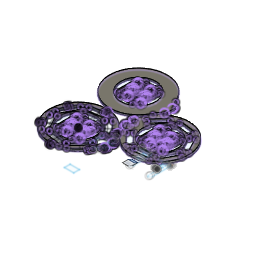
plywood_lamp (Autodesk Fusion 360 design; units mm, degrees)
Autodesk Fusion 360 part; units mm, degrees
(part 1 of 2)
sketch "Sketch1" plane through (0, 0, 0) normal (0, 1, 0) x (1, 0, 0)
  circle A0 centre (0, 0) radius 32
  circle A1 centre (0, 0) radius 52.5
  line L0 (34, 9.25) -> (57, 9.25)
  line L1 (57, 9.25) -> (57, -9.25)
  line L2 (57, -9.25) -> (34, -9.25)
  line L3 (34, -9.25) -> (34, 9.25)
  line L4 (50, 4.3983) -> (59, 4.3983)
  line L5 (59, 4.3983) -> (59, -4.6017)
  line L6 (59, -4.6017) -> (50, -4.6017)
  line L7 (50, -4.6017) -> (50, 4.3983)
  line L8 (50, -65) -> (67, -65)
  line L9 (67, -65) -> (67, -75.4)
  line L10 (67, -75.4) -> (50, -75.4)
  line L11 (50, -75.4) -> (50, -65)
  line L12 (0, 0) -> (34, 0)
  line L13 (0, 0) -> (25.0674, -22.9701)
  line L14 (25.0674, -22.9701) -> (36.5525, -10.4364)
  line L15 (36.5525, -10.4364) -> (44.2201, -17.4625)
  line L16 (44.2201, -17.4625) -> (32.7351, -29.9962)
  line L17 (32.7351, -29.9962) -> (25.0674, -22.9701)
  line L18 (25.0674, -22.9701) -> (13.5824, -35.5038)
  line L19 (13.5824, -35.5038) -> (21.2501, -42.5299)
  line L20 (21.2501, -42.5299) -> (32.7351, -29.9962)
  line L21 (32.7351, -29.9962) -> (25.0674, -22.9701)
  line L22 (0, 0) -> (-4.4379, -33.7091)
  line L23 (-5.7954, -44.0202) -> (-4.4379, -33.7091)
  line L24 (-4.4379, -33.7091) -> (12.4167, -35.9281)
  line L25 (11.0592, -46.2391) -> (-5.7954, -44.0202)
  line L26 (12.4167, -35.9281) -> (11.0592, -46.2391)
  line L27 (-4.4379, -33.7091) -> (-21.2925, -31.4902)
  line L28 (-22.6499, -41.8012) -> (-5.7954, -44.0202)
  line L29 (-21.2925, -31.4902) -> (-22.6499, -41.8012)
  line L30 (0, 0) -> (-30.1584, -15.6995)
  line L31 (-39.3833, -20.5016) -> (-30.1584, -15.6995)
  line L32 (-30.1584, -15.6995) -> (-22.3086, -30.7786)
  line L33 (-31.5336, -35.5808) -> (-39.3833, -20.5016)
  line L34 (-22.3086, -30.7786) -> (-31.5336, -35.5808)
  line L35 (-30.1584, -15.6995) -> (-38.0081, -0.6203)
  line L36 (-47.233, -5.4225) -> (-39.3833, -20.5016)
  line L37 (-38.0081, -0.6203) -> (-47.233, -5.4225)
  line L38 (0, 0) -> (-30.1584, 15.6995)
  line L39 (-39.3833, 20.5016) -> (-30.1584, 15.6995)
  line L40 (-30.1584, 15.6995) -> (-38.0081, 0.6203)
  line L41 (-47.233, 5.4225) -> (-39.3833, 20.5016)
  line L42 (-38.0081, 0.6203) -> (-47.233, 5.4225)
  line L43 (-30.1584, 15.6995) -> (-22.3086, 30.7786)
  line L44 (-31.5336, 35.5808) -> (-39.3833, 20.5016)
  line L45 (-22.3086, 30.7786) -> (-31.5336, 35.5808)
  line L46 (0, 0) -> (-4.4379, 33.7091)
  line L47 (-5.7954, 44.0202) -> (-4.4379, 33.7091)
  line L48 (-4.4379, 33.7091) -> (-21.2925, 31.4902)
  line L49 (-22.6499, 41.8012) -> (-5.7954, 44.0202)
  line L50 (-21.2925, 31.4902) -> (-22.6499, 41.8012)
  line L51 (-4.4379, 33.7091) -> (12.4167, 35.9281)
  line L52 (11.0592, 46.2391) -> (-5.7954, 44.0202)
  line L53 (12.4167, 35.9281) -> (11.0592, 46.2391)
  line L54 (0, 0) -> (25.0674, 22.9701)
  line L55 (32.7351, 29.9962) -> (25.0674, 22.9701)
  line L56 (25.0674, 22.9701) -> (13.5824, 35.5038)
  line L57 (21.2501, 42.5299) -> (32.7351, 29.9962)
  line L58 (13.5824, 35.5038) -> (21.2501, 42.5299)
  line L59 (25.0674, 22.9701) -> (36.5525, 10.4364)
  line L60 (44.2201, 17.4625) -> (32.7351, 29.9962)
  line L61 (36.5525, 10.4364) -> (44.2201, 17.4625)
  circle A2 centre (0, 0) radius 38.0132
  circle A3 centre (0, 0) radius 47.5432
  line L62 (55, 12.25) -> (34, 12.25)
  line L63 (34, 12.25) -> (34, -12.25)
  line L64 (34, -12.25) -> (55, -12.25)
  line L65 (60, -7.25) -> (60, 7.25)
  arc A4 (55, -12.25) -> (60, -7.25) centre (55, -7.25) ccw
  arc A5 (60, 7.25) -> (55, 12.25) centre (55, 7.25) ccw
  spline S0 degree 5 poles (58.5355, -10.7855) (58.375, -10.946) (58.0274, -11.2549) (57.426, -11.6816) (56.4828, -12.1897) (55.1674, -12.7909) (53.8333, -13.4415) (52.5876, -14.2222) (51.4896, -15.1867) (50.5348, -16.3509) (49.6862, -17.7123) (49.0515, -18.9501) (48.5799, -19.957) (48.2645, -20.6625) (48.1066, -21.0238) knots 0 0 0 0 0 0 0.1 0.2 0.3 0.4 0.5 0.6 0.7 0.8 0.9 1 1 1 1 1 1
  line L66 (59.4934, -9.8277) -> (57.5777, -11.7434)
  line L67 (48.9119, -19.1812) -> (47.3014, -22.8664)
  spline S1 degree 5 poles (58.5355, 10.7855) (58.3764, 10.9446) (58.0317, 11.2507) (57.4349, 11.6734) (56.4973, 12.1769) (55.1846, 12.7765) (53.845, 13.4321) (52.5838, 14.2253) (51.463, 15.2079) (50.4859, 16.3894) (49.6261, 17.7595) (48.9998, 18.9905) (48.5482, 19.9817) (48.2529, 20.6716) (48.1066, 21.0238) knots 0 0 0 0 0 0 0.1 0.2 0.3 0.4 0.5 0.6 0.7 0.8 0.9 1 1 1 1 1 1
  line L68 (59.4849, 9.8361) -> (57.5861, 11.7349)
  line L69 (48.851, 19.231) -> (47.3623, 22.8167)
  spline S2 degree 5 poles (57, -9.25) (56.1534, -9.25) (54.5378, -9.3901) (52.3465, -10.0199) (49.8421, -11.547) (47.2933, -13.9608) (45.7147, -15.761) (44.8358, -16.7778) (44.4003, -17.2659) (44.2201, -17.4625) knots 0 0 0 0 0 0 0.2 0.4 0.6 0.8 1 1 1 1 1 1
  line L70 (59, -9.25) -> (55, -9.25)
  line L71 (44.672, -16.9694) -> (43.7683, -17.9556)
  spline S3 degree 5 poles (57, 9.25) (56.1534, 9.25) (54.557, 9.3691) (52.452, 9.9048) (50.1458, 11.2155) (47.8255, 13.38) (46.2557, 15.1706) (45.1945, 16.3864) (44.5366, 17.1171) (44.2201, 17.4625) knots 0 0 0 0 0 0 0.2 0.4 0.6 0.8 1 1 1 1 1 1
  line L72 (59, 9.25) -> (55, 9.25)
  line L73 (45.0141, 16.5961) -> (43.4262, 18.3289)
  line L74 (59, 4.3983) -> (60, 4.3983)
  line L75 (59, -4.6017) -> (60, -4.6017)
  line L76 (0, 0) -> (45.4663, -26.25)
  line L77 (41.1362, -23.75) -> (42.0112, -22.2345)
  line L78 (42.0112, -22.2345) -> (46.3161, -24.7199)
  line L79 (41.1362, -23.75) -> (40.2612, -25.2655)
  line L80 (40.2612, -25.2655) -> (44.5661, -27.751)
  line L81 (0, 0) -> (45.4663, 26.25)
  line L82 (40.2612, 25.2655) -> (44.5661, 27.751)
  line L83 (42.0112, 22.2345) -> (46.3161, 24.7199)
  line L84 (41.1362, 23.75) -> (42.0112, 22.2345)
  line L85 (41.1362, 23.75) -> (40.2612, 25.2655)
  line L86 (0, 0) -> (0, 52.5)
  line L87 (-1.75, 47.5) -> (-1.75, 52.4708)
  line L88 (1.75, 47.5) -> (1.75, 52.4708)
  line L89 (0, 47.5) -> (1.75, 47.5)
  line L90 (0, 47.5) -> (-1.75, 47.5)
  line L91 (0, 0) -> (-45.4663, 26.25)
  line L92 (-42.0112, 22.2345) -> (-46.3161, 24.7199)
  line L93 (-40.2612, 25.2655) -> (-44.5661, 27.751)
  line L94 (-41.1362, 23.75) -> (-40.2612, 25.2655)
  line L95 (-41.1362, 23.75) -> (-42.0112, 22.2345)
  line L96 (0, 0) -> (-45.4663, -26.25)
  line L97 (-40.2612, -25.2655) -> (-44.5661, -27.751)
  line L98 (-42.0112, -22.2345) -> (-46.3161, -24.7199)
  line L99 (-41.1362, -23.75) -> (-42.0112, -22.2345)
  line L100 (-41.1362, -23.75) -> (-40.2612, -25.2655)
  line L101 (0, 0) -> (0, -52.5)
  line L102 (1.75, -47.5) -> (1.75, -52.4708)
  line L103 (-1.75, -47.5) -> (-1.75, -52.4708)
  line L104 (0, -47.5) -> (-1.75, -47.5)
  line L105 (0, -47.5) -> (1.75, -47.5)
  line L106 (100, 19.5) -> (105, 19.5)
  line L107 (105, 19.5) -> (105, 23)
  line L108 (105, 23) -> (90, 23)
  line L109 (100, 19.5) -> (100, 15)
  line L110 (100, 15) -> (105, 15)
  line L111 (105, 15) -> (105, 11.5)
  line L112 (105, 11.5) -> (98.5, 11.5)
  line L113 (90, 23) -> (90, 28) construction
  line L114 (90, 28) -> (100, 28) construction
  spline S4 degree 2 poles (90, 23) (90, 28) (100, 28) knots 0 0 0 1 1 1
  line L115 (110, 23) -> (110, 28) construction
  line L116 (110, 28) -> (100, 28) construction
  spline S5 degree 2 poles (110, 23) (110, 28) (100, 28) knots 0 0 0 1 1 1
  line L117 (104.8291, 6) -> (104.8291, -12.0001)
  arc A6 (104.8291, 6) -> (103.8291, 7) centre (103.8291, 6) ccw
  arc A7 (104.8291, -12.0001) -> (105.8149, -13) centre (105.8291, -12.0001) ccw
  line L118 (25.4361, -23.3079) -> (14.9644, -34.7357)
  line L119 (14.9644, -34.7357) -> (21.8948, -41.0862)
  line L120 (21.8948, -41.0862) -> (42.8381, -18.2306)
  line L121 (42.8381, -18.2306) -> (35.9077, -11.8801)
  line L122 (35.9077, -11.8801) -> (25.4361, -23.3079)
  line L123 (-21.0975, -41.5013) -> (9.6373, -45.5476)
  line L124 (-4.5032, -34.2048) -> (-19.8705, -32.1817)
  line L125 (10.8642, -36.228) -> (-4.5032, -34.2048)
  line L126 (-19.8705, -32.1817) -> (-21.0975, -41.5013)
  line L127 (9.6373, -45.5476) -> (10.8642, -36.228)
  line L128 (-46.0969, -6.5221) -> (-31.7827, -34.0194)
  line L129 (-30.6019, -15.9303) -> (-37.759, -2.1817)
  line L130 (-23.4448, -29.679) -> (-30.6019, -15.9303)
  line L131 (-37.759, -2.1817) -> (-46.0969, -6.5221)
  line L132 (-31.7827, -34.0194) -> (-23.4448, -29.679)
  line L133 (-31.7827, 34.0194) -> (-46.0969, 6.5221)
  line L134 (-30.6019, 15.9303) -> (-23.4448, 29.679)
  line L135 (-37.759, 2.1817) -> (-30.6019, 15.9303)
  line L136 (-23.4448, 29.679) -> (-31.7827, 34.0194)
  line L137 (-46.0969, 6.5221) -> (-37.759, 2.1817)
  line L138 (9.6373, 45.5476) -> (-21.0975, 41.5013)
  line L139 (-4.5032, 34.2048) -> (10.8642, 36.228)
  line L140 (-19.8705, 32.1817) -> (-4.5032, 34.2048)
  line L141 (10.8642, 36.228) -> (9.6373, 45.5476)
  line L142 (-21.0975, 41.5013) -> (-19.8705, 32.1817)
  line L143 (42.8381, 18.2306) -> (21.8948, 41.0862)
  line L144 (25.4361, 23.3079) -> (35.9077, 11.8801)
  line L145 (14.9644, 34.7357) -> (25.4361, 23.3079)
  line L146 (35.9077, 11.8801) -> (42.8381, 18.2306)
  line L147 (21.8948, 41.0862) -> (14.9644, 34.7357)
  line L148 (110, 23) -> (110, -9)
  line L149 (106, -13) -> (105.8149, -13)
  arc A8 (106, -13) -> (110, -9) centre (106, -9) ccw
  line L150 (103.8291, 7) -> (103, 7)
  arc A9 (98.5, 11.5) -> (103, 7) centre (103, 11.5) ccw
  line L151 (135, 19.5) -> (135, 15)
  spline S6 degree 2 poles (145, 23) (145, 28) (135, 28) knots 0 0 0 1 1 1
  line L152 (145, 23) -> (145, 28) construction
  line L153 (145, 28) -> (135, 28) construction
  line L154 (140, 23) -> (125, 23)
  line L155 (140, 15) -> (140, 11.5)
  line L156 (145, 23) -> (145, -9)
  arc A10 (141, -13) -> (145, -9) centre (141, -9) ccw
  line L157 (141, -13) -> (140.8149, -13)
  line L158 (135, 19.5) -> (140, 19.5)
  line L159 (135, 15) -> (140, 15)
  spline S7 degree 2 poles (125, 23) (125, 28) (135, 28) knots 0 0 0 1 1 1
  line L160 (125, 23) -> (125, 28) construction
  line L161 (125, 28) -> (135, 28) construction
  line L162 (140, 19.5) -> (140, 23)
  line L163 (140, 11.5) -> (132.5, 11.5)
  line L164 (139.3, 5.7) -> (139.3, -11.5)
  line L165 (132.5, 11.5) -> (132.5, 7.5)
  line L166 (133, 7) -> (138, 7)
  arc A11 (132.5, 7.5) -> (133, 7) centre (133, 7.5) ccw
  line L167 (133, 7) -> (133.5, 7) construction
  line L168 (133.5, 7) -> (133.5, 7.5) construction
  line L169 (133.5, 7.5) -> (135.5, 7.5) construction
  line L170 (135.5, 7.5) -> (137.5, 7.5) construction
  line L171 (137.5, 7.5) -> (137.5, 7) construction
  line L172 (137.5, 7) -> (138, 7) construction
  spline S8 degree 5 poles (133, 7) (133.5, 7) (133.5, 7.5) (135.5, 7.5) (137.5, 7.5) (137.5, 7) (138, 7) knots 0 0 0 0 0 0 0.5 1 1 1 1 1 1
  arc A12 (139.3, 5.7) -> (138, 7) centre (138, 5.7) ccw
  line L173 (140.8, -13) -> (140.8149, -13)
  arc A13 (139.3, -11.5) -> (140.8, -13) centre (140.8, -11.5) ccw
  point P0 (53, -14)
  point P1 (53, 14)
  dimension "d1" = 23
  dimension "d2" = 18.5
  dimension "d3" = 64
  dimension "d4" = 105
  dimension "d5" = 9
  dimension "d6" = 2
  dimension "d7" = 9
  dimension "d8" = 9.25
  dimension "d9" = 34
  dimension "d10" = 17
  dimension "d11" = 10.4
  dimension "d14" = 42.5
  dimension "d15" = 34
  dimension "d16" = 17
  dimension "d17" = 10.4
  dimension "d18" = 17
  dimension "d19" = 10.4
  dimension "d21" = -275
  dimension "d22" = 3
  dimension "d23" = 3
  dimension "d24" = 3
  dimension "d25" = 5
  dimension "d26" = 5
  dimension "d29" = 30
  dimension "d30" = 5
  dimension "d31" = 1.75
  dimension "d32" = 1.75
  dimension "d34" = 360
  dimension "d35" = 15
  dimension "d37" = 3.5
  dimension "d38" = 5
  dimension "d41" = 4.5
  dimension "d42" = 5
  dimension "d43" = 3.5
  dimension "d44" = 6.5
  dimension "d46" = 5
  dimension "d47" = 10
  dimension "d49" = 1
  dimension "d50" = 1
  dimension "d52" = 0.5
  dimension "d53" = 0.5
  dimension "d54" = 1.5
  dimension "d55" = 1.5
  dimension "d57" = -275
  dimension "d76" = 5
  dimension "d77" = 4
  dimension "d78" = 4.5
  dimension "d87" = 15
  dimension "d88" = 3.5
  dimension "d89" = 5
  dimension "d90" = 4.5
  dimension "d91" = 5
  dimension "d92" = 3.5
  dimension "d93" = 7.5
  dimension "d94" = 5
  dimension "d95" = 10
  dimension "d98" = 5
  dimension "d99" = 4
  dimension "d103" = 0.7
  dimension "d104" = 4.5
  dimension "d105" = 0.5
  dimension "d106" = 1.3
  dimension "d107" = 1.5
  constraint coincident A0.centre A1.centre
  constraint concentric A0 A1
  constraint horizontal L0
  constraint vertical L1
  constraint horizontal L2
  constraint vertical L3
  constraint horizontal L4
  constraint vertical L5
  constraint horizontal L6
  constraint vertical L7
  constraint horizontal L8
  constraint vertical L9
  constraint horizontal L10
  constraint vertical L11
  constraint midpoint L3 L12.end
  constraint perpendicular L13 L14
  constraint perpendicular L14 L15
  constraint perpendicular L14 L17
  constraint perpendicular L13 L18
  constraint perpendicular L18 L19
  constraint perpendicular L20 L21
  constraint perpendicular L16 L17
  constraint coincident L18.end A2
  constraint coincident L25.start A3
  constraint horizontal L62
  constraint vertical L63
  constraint horizontal L64
  constraint vertical L65
  constraint tangent L64 A4
  constraint tangent L65 A4
  constraint tangent L62 A5
  constraint tangent L65 A5
  constraint midpoint A4 S0.start
  constraint coincident A1 S0.end
  constraint midpoint S0.start L66
  constraint tangent A4 L66
  constraint midpoint S0.end L67
  constraint tangent A1 L67
  constraint midpoint A5 S1.start
  constraint coincident A1 S1.end
  constraint midpoint S1.start L68
  constraint tangent A5 L68
  constraint midpoint S1.end L69
  constraint coincident A1 L69.start
  constraint midpoint L1.end L70
  constraint coincident L2 L70.end
  constraint midpoint L15.end L71
  constraint coincident L16 L71.end
  constraint midpoint L0.end L72
  constraint coincident L0 L72.end
  constraint midpoint L60.start L73
  constraint coincident L60 L73.end
  constraint coincident L65 L74.end
  constraint perpendicular L65 L74
  constraint coincident L65 L75.end
  constraint perpendicular L65 L75
  constraint coincident A1 L76.end
  constraint coincident L76 L77.start
  constraint perpendicular L76 L77
  constraint coincident A1 L78.end
  constraint perpendicular L77 L78
  constraint perpendicular L76 L79
  constraint coincident A1 L80.end
  constraint perpendicular L79 L80
  constraint horizontal L106
  constraint perpendicular L106 L107
  constraint perpendicular L1 L108
  constraint perpendicular L106 L109
  constraint perpendicular L109 L110
  constraint perpendicular L106 L111
  constraint perpendicular L111 L112
  constraint parallel L108 L116
  constraint parallel L108 L114
  constraint parallel L113 L115
  constraint perpendicular L108 L113
  constraint perpendicular L112 L117
  constraint tangent L117 A6
  constraint tangent L117 A7
  constraint coincident L17 L118.start
  constraint perpendicular L21 L118
  constraint perpendicular L118 L119
  constraint perpendicular L21 L120
  constraint perpendicular L16 L121
  constraint collinear L118 L122
  constraint tangent L148 A8
  constraint tangent L149 A8
  constraint tangent L150 A9
  constraint coincident L112.end A9.start
  constraint horizontal L158
  constraint perpendicular L158 L162
  constraint perpendicular L151 L158
  constraint perpendicular L151 L159
  constraint perpendicular L155 L158
  constraint perpendicular L155 L163
  constraint parallel L153 L154
  constraint parallel L154 L161
  constraint parallel L152 L160
  constraint perpendicular L154 L160
  constraint tangent L156 A10
  constraint tangent A10 L157
  constraint vertical L164
  constraint perpendicular L163 L165
  constraint perpendicular L164 L166
  constraint tangent L165 A11
  constraint tangent L166 A11
  constraint coincident L166 L167.end
  constraint coincident L166 L171.end
  constraint coincident L166 L172.end
  constraint tangent L164 A12
  constraint tangent L166 A12
  constraint tangent L164 A13
  constraint tangent L173 A13
  measures "d1" distance of L0.start L0.end
  measures "d2" distance of L0.end L1.end
  measures "d3" diameter of A0
  measures "d4" diameter of A1
  measures "d5" distance of L4.start L4.end
  measures "d6" distance of L1 L5
  measures "d7" distance of L4 L6
  measures "d8" distance of A0.centre L2
  measures "d9" distance of A0.centre L3
  measures "d10" distance of L8.start L8.end
  measures "d11" distance of L8.end L9.end
  measures "d14" angle of L12 L13
  measures "d15" distance of A0.centre L13.end
  measures "d16" distance of L13.end L14.end
  measures "d17" distance of L14.end L15.end
  measures "d18" distance of L13.end L18.end
  measures "d19" distance of L18.end L19.end
  measures "d22" distance of L0 L62
  measures "d23" distance of L2 L64
  measures "d24" distance of L1 L65
  measures "d25" radius of A4 L15
  measures "d26" radius of A5 L15
  measures "d29" angle of L12 L76
  measures "d30" distance of L76.end L77.start
  measures "d31" distance of L76 L78
  measures "d32" distance of L76 L80
  measures "d35" distance of L107.end L108.end
  measures "d37" distance of L106.end L107.end
  measures "d38" distance of L106.start L106.end
  measures "d41" distance of L106.start L109.end
  measures "d42" distance of L109.end L110.end
  measures "d43" distance of L110.end L111.end
  measures "d44" distance of L111.end L112.end
  measures "d46" distance of L108 L114.end
  measures "d47" distance of L114.end L115.end
  measures "d49" radius of A6
  measures "d50" radius of A7
  measures "d52" distance of L18 L118
  measures "d53" distance of L20 L120
  measures "d54" distance of L19 L119
  measures "d55" distance of L15 L121
  measures "d76" distance of L115.start L115.end
  measures "d77" radius of A8
  measures "d78" radius of A9
  measures "d87" distance of L154.start L154.end
  measures "d88" distance of L158.end L154.start
  measures "d89" distance of L151.start L158.end
  measures "d90" distance of L151.start L151.end
  measures "d91" distance of L155.start L151.end
  measures "d92" distance of L155.start L155.end
  measures "d93" distance of L155.end L163.end
  measures "d94" distance of S6.end L154
  measures "d95" distance of L152.end S6.end
  measures "d98" distance of L152.end S6.start
  measures "d99" radius of A10
  measures "d103" distance of L155 L164
  measures "d104" distance of L163 L166
  measures "d105" radius of A11
  measures "d106" radius of A12
  measures "d107" radius of A13
extrude "Extrude9" add sketch "Sketch1" along normal blind 3 contours A0 L3 L12 L14 L63 L64 L76 | A0 L3 L12 L59 L62 L63 L81 | A0 L54 L59 L81 | A0 L13 L14 L76 | L0 L2 L3 A2 L63 | A0 L51 L54 L56 A2 L86 | L59 L62 L81 L144 | L55 L59 L81 L144 | A0 L13 L18 L24 A2 L101 | L14 L17 L21 L76 L122 | L14 L64 L76 L122 | A0 L22 L27 L32 A2 L96 | A0 L22 L24 L101 | A0 L30 L35 L38 L40 A2 | A0 L30 L32 L96 | A0 L38 L43 L91 | A0 L46 L51 L86 | A0 L43 L46 L48 A2 L91 | L2 L14 A2 L63 L64 | L0 L59 A2 L62 L63 | L55 L56 A2 L145 L147 | L59 A2 L62 L144 L146 | L55 A2 L81 L144 | A2 L62 L81 L144 | L17 L18 L21 A2 L118 L119 | L14 A2 L64 L121 L122 | A2 L64 L76 L122 | L17 L21 A2 L76 L122 | L23 L24 L101 L125 | L23 L27 A2 L124 L126 | L31 L32 L96 L130 | L31 L35 A2 L129 L131 | L39 L40 A2 L135 L137 | L39 L43 L91 L134 | L47 L48 A2 L140 L142 | L47 L51 L86 L139 | L51 A2 L86 L139 L141 | L43 A2 L91 L134 L136 | L32 A2 L96 L130 L132 | L24 A2 L101 L125 L127 | L0 L2 A2 A3 | L2 L15 A2 A3 L64 | L0 L61 A2 A3 L62 | L55 A2 L145 L147 | L53 L58 A2 A3 | L55 L57 L58 A2 L143 L147 | L61 A2 L62 L146 | A2 L62 L144 L146 | A2 L62 L81 L143 L146 | L55 A2 L81 L143 | L17 L21 A2 L118 L119 | L17 L19 L20 L21 A2 L119 L120 | L19 L26 A2 A3 | L15 A2 L64 L121 | A2 L64 L121 L122 | L17 L21 A2 L76 L120 | A2 L64 L76 L120 L121 | L23 A2 L101 L125 | L23 A2 L124 L126 | L23 L28 L29 A2 L123 L126 | L29 L34 A2 A3 | L31 A2 L96 L130 | L31 A2 L129 L131 | L31 L36 L37 A2 L128 L131 | L37 L42 A2 A3 | L39 A2 L135 L137 | L39 A2 L91 L134 | L39 L41 L42 A2 L133 L137 | L47 A2 L140 L142 | L47 A2 L86 L139 | L45 L50 A2 A3 | L47 L49 L50 A2 L138 L142 | L52 L53 A2 L86 L138 L141 | A2 L86 L139 L141 | L44 L45 A2 L91 L133 L136 | A2 L91 L134 L136 | L33 L34 A2 L96 L128 L132 | A2 L96 L130 L132 | L25 L26 A2 L101 L123 L127 | A2 L101 L125 L127 | A1 L0 L2 L4 L6 L7 A3 | A1 L2 A3 L64 S2 | A1 L0 A3 L62 S3 | L55 A2 L143 L147 | L57 L60 A3 L81 L82 L85 | A1 A3 L82 L88 | L60 L61 L62 L73 L81 L143 L146 | L61 A3 L62 | A2 L62 L146 | L55 L60 L81 L143 | L17 L21 A2 L119 L120 | A1 A3 L80 L102 | L16 L20 A3 L76 L79 L80 | L15 A3 L64 | L15 L16 L64 L71 L76 L120 L121 | A2 L64 L121 | L16 L17 L21 L76 L120 | L23 A2 L101 L123 | L23 A2 L123 L126 | A1 A3 L97 L103 | L25 L28 A3 L101 L103 L104 | L31 A2 L96 L128 | L31 A2 L128 L131 | A1 A3 L92 L98 | L33 L36 A3 L96 L98 L99 | L39 A2 L133 L137 | L39 A2 L91 L133 | L41 L44 A3 L91 L92 L95 | L47 A2 L138 L142 | L47 A2 L86 L138 | L49 L52 A3 L86 L87 L90 | A1 A3 L87 L93 | L52 A3 L86 L88 L89 | A2 L86 L138 L141 | L44 A3 L91 L93 L94 | A2 L91 L133 L136 | L33 A3 L96 L97 L100 | A2 L96 L128 L132 | L25 A3 L101 L102 L105 | A2 L101 L123 L127 | A1 L2 S2 L70 | A1 L1 L2 L6 L70 | A3 L64 S2 | A1 L0 L1 L4 L72 | A1 L0 S3 L72 | A3 L62 S3 | A1 A3 L81 L82 | A3 L81 L82 L85 | L60 A3 L73 L81 L83 L84 | A1 A3 L62 L69 S3 L83 | A3 L76 L79 L80 | A1 A3 L76 L80 | L16 A3 L71 L76 L77 L78 | A1 A3 L64 S2 L78 | L23 L25 L101 L123 | A3 L101 L103 L104 | A1 A3 L101 L103 | L31 L33 L96 L128 | A3 L96 L98 L99 | A1 A3 L96 L98 | L39 L44 L91 L133 | A1 A3 L91 L92 | A3 L91 L92 L95 | L47 L52 L86 L138 | A1 A3 L86 L87 | A3 L86 L87 L90 | A3 L86 L88 L89 | A1 A3 L86 L88 | A3 L91 L93 L94 | A1 A3 L91 L93 | A1 A3 L96 L97 | A3 L96 L97 L100 | A1 A3 L101 L102 | A3 L101 L102 L105 | A1 L1 L4 L62 L65 A5 S3 L74 | A1 L1 L6 L64 L65 A4 S2 L75 | A1 L64 S2 | A1 L4 L6 L7 | A1 L1 L4 L6 | A1 L62 S3 | A1 A3 L81 L83 | A3 L81 L83 L84 | A3 L76 L77 L78 | A1 A3 L76 L78 | A1 L64 A4 S0 | L1 L4 L5 L6 | A1 L62 A5 S1 | L5 L65 L74 L75 | A1 S1 L69 | A1 S1 makes body 1
move_body "Move25" bodies 1 to x (1, 0, 0) y (0, 1, 0) z (0, 0, 1) at (0, 0, -110)
extrude "Extrude10" add sketch "Sketch1" along normal blind 4 separate body contours A0 L3 L12 L14 L63 L64 L76 | A0 L3 L12 L59 L62 L63 L81 | A0 L54 L59 L81 | A0 L13 L14 L76 | L0 L2 L3 A2 L63 | A0 L51 L54 L56 A2 L86 | L59 L62 L81 L144 | L55 L59 L81 L144 | A0 L13 L18 L24 A2 L101 | L14 L17 L21 L76 L122 | L14 L64 L76 L122 | A0 L22 L27 L32 A2 L96 | A0 L22 L24 L101 | A0 L30 L35 L38 L40 A2 | A0 L30 L32 L96 | A0 L38 L43 L91 | A0 L46 L51 L86 | A0 L43 L46 L48 A2 L91 | L2 L14 A2 L63 L64 | L0 L59 A2 L62 L63 | L55 L56 A2 L145 L147 | L59 A2 L62 L144 L146 | L17 L18 L21 A2 L118 L119 | L14 A2 L64 L121 L122 | L23 L24 L101 L125 | L23 L27 A2 L124 L126 | L31 L32 L96 L130 | L31 L35 A2 L129 L131 | L39 L40 A2 L135 L137 | L39 L43 L91 L134 | L47 L48 A2 L140 L142 | L47 L51 L86 L139 | L51 A2 L86 L139 L141 | L43 A2 L91 L134 L136 | L32 A2 L96 L130 L132 | L24 A2 L101 L125 L127 | L0 L2 A2 A3 | L2 L15 A2 A3 L64 | L0 L61 A2 A3 L62 | L53 L58 A2 A3 | L55 L57 L58 A2 L143 L147 | L61 A2 L62 L146 | L17 L19 L20 L21 A2 L119 L120 | L19 L26 A2 A3 | L15 A2 L64 L121 | L23 L28 L29 A2 L123 L126 | L29 L34 A2 A3 | L31 L36 L37 A2 L128 L131 | L37 L42 A2 A3 | L39 L41 L42 A2 L133 L137 | L45 L50 A2 A3 | L47 L49 L50 A2 L138 L142 | L52 L53 A2 L86 L138 L141 | L44 L45 A2 L91 L133 L136 | L33 L34 A2 L96 L128 L132 | L25 L26 A2 L101 L123 L127 | A1 L0 L2 L4 L6 L7 A3 | A1 L2 A3 L64 S2 | A1 L0 A3 L62 S3 | L57 L60 A3 L81 L82 L85 | A1 A3 L82 L88 | L60 L61 L62 L73 L81 L143 L146 | L61 A3 L62 | L55 L60 L81 L143 | A1 A3 L80 L102 | L16 L20 A3 L76 L79 L80 | L15 A3 L64 | L15 L16 L64 L71 L76 L120 L121 | L16 L17 L21 L76 L120 | A1 A3 L97 L103 | L25 L28 A3 L101 L103 L104 | A1 A3 L92 L98 | L33 L36 A3 L96 L98 L99 | L41 L44 A3 L91 L92 L95 | L49 L52 A3 L86 L87 L90 | A1 A3 L87 L93 | L52 A3 L86 L88 L89 | L44 A3 L91 L93 L94 | L33 A3 L96 L97 L100 | L25 A3 L101 L102 L105 | A1 L2 S2 L70 | A1 L1 L2 L6 L70 | A3 L64 S2 | A1 L0 L1 L4 L72 | A1 L0 S3 L72 | A3 L62 S3 | A1 A3 L81 L82 | A3 L81 L82 L85 | L60 A3 L73 L81 L83 L84 | A1 A3 L62 L69 S3 L83 | A3 L76 L79 L80 | A1 A3 L76 L80 | L16 A3 L71 L76 L77 L78 | A1 A3 L64 S2 L78 | L23 L25 L101 L123 | A3 L101 L103 L104 | A1 A3 L101 L103 | L31 L33 L96 L128 | A3 L96 L98 L99 | A1 A3 L96 L98 | L39 L44 L91 L133 | A1 A3 L91 L92 | A3 L91 L92 L95 | L47 L52 L86 L138 | A1 A3 L86 L87 | A3 L86 L87 L90 | A3 L86 L88 L89 | A1 A3 L86 L88 | A3 L91 L93 L94 | A1 A3 L91 L93 | A1 A3 L96 L97 | A3 L96 L97 L100 | A1 A3 L101 L102 | A3 L101 L102 L105 | A1 L1 L4 L62 L65 A5 S3 L74 | A1 L1 L6 L64 L65 A4 S2 L75 | A1 L64 S2 | A1 L62 S3 | A1 A3 L81 L83 | A3 L81 L83 L84 | A3 L76 L77 L78 | A1 A3 L76 L78 | A1 L64 A4 S0 | A1 L62 A5 S1 | A1 S1 L69 | A1 S1 makes body 2
move_body "Move26" bodies 2 to x (1, 0, 0) y (0, 1, 0) z (0, 0, 1) at (0, 0, 110)
extrude "Extrude11" add sketch "Sketch1" along normal blind 4 separate body contours A0 L3 L12 L14 L63 L64 L76 | A0 L3 L12 L59 L62 L63 L81 | A0 L54 L59 L81 | A0 L13 L14 L76 | A0 L51 L54 L56 A2 L86 | A0 L13 L18 L24 A2 L101 | A0 L22 L27 L32 A2 L96 | A0 L22 L24 L101 | A0 L30 L35 L38 L40 A2 | A0 L30 L32 L96 | A0 L38 L43 L91 | A0 L46 L51 L86 | A0 L43 L46 L48 A2 L91 | L2 L14 A2 L63 L64 | L0 L59 A2 L62 L63 | L59 A2 L62 L144 L146 | L0 L61 A2 A3 L62 | L61 A2 L62 L146 | A2 L62 L144 L146 | A1 L0 A3 L62 S3 | L57 L60 A3 L81 L82 L85 | A1 A3 L82 L88 | L61 A3 L62 | A2 L62 L146 | A1 A3 L80 L102 | L16 L20 A3 L76 L79 L80 | A1 A3 L97 L103 | L25 L28 A3 L101 L103 L104 | A1 A3 L92 L98 | L33 L36 A3 L96 L98 L99 | L41 L44 A3 L91 L92 L95 | L49 L52 A3 L86 L87 L90 | A1 A3 L87 L93 | L52 A3 L86 L88 L89 | L44 A3 L91 L93 L94 | L33 A3 L96 L97 L100 | L25 A3 L101 L102 L105 | A1 L0 S3 L72 | A3 L62 S3 | A3 L81 L82 L85 | L60 A3 L73 L81 L83 L84 | A1 A3 L62 L69 S3 L83 | A3 L76 L79 L80 | L16 A3 L71 L76 L77 L78 | A1 A3 L64 S2 L78 | A3 L101 L103 L104 | A3 L96 L98 L99 | A3 L91 L92 L95 | A3 L86 L87 L90 | A3 L86 L88 L89 | A3 L91 L93 L94 | A3 L96 L97 L100 | A3 L101 L102 L105 | A1 L1 L4 L62 L65 A5 S3 L74 | A1 L1 L6 L64 L65 A4 S2 L75 | A1 L64 S2 | A1 L62 S3 | A3 L81 L83 L84 | A3 L76 L77 L78 | A1 L64 A4 S0 | A1 L62 A5 S1 | A1 S1 L69 | A1 S1 makes body 3
move_body "Move41" bodies 2 to x (1, 0, 0) y (0, 1, 0) z (0, 0, 1) at (140, 0, 0)
extrude "Extrude13" add sketch "Sketch1" along normal blind 4 separate body contours L151 S6 L154 L155 L156 A10 L157 L158 L159 S7 L162 L163 L164 L165 A11 S8 A12 L173 A13 makes body 4
copy_body "CopyPasteBodies10" bodies 4 makes body 5
move_body "Move42" bodies 5 to x (-1, 0, 0) y (0, 1, 0) z (0, 0, -1) at (270, 0, -9)
copy_body "CopyPasteBodies11" bodies 4 5 makes body 6 makes body 7
move_body "Move43" bodies 6 7 to x (1, 0, 0) y (0, 1, 0) z (0, 0, 1) at (23, 0, 0)
move_body "Move44" bodies 6 7 5 4 to x (1, 0, 0) y (0, 1, 0) z (0, 0, 1) at (85, 0, -51.5)
move_body "Move45" bodies 7 6 5 4 to x (1, 0, 0) y (0, 1, 0) z (0, 0, 1) at (1, 0, 0)
move_body "Move47" bodies 2 to x (-1, 0, 0) y (0, 1, 0) z (0, 0, -1) at (235, 0, 55)
copy_body "CopyPasteBodies13" bodies 7 6 5 4 makes body 8 makes body 9 makes body 10 makes body 11
move_body "Move48" bodies 8 9 10 11 to x (1, 0, 0) y (0, 1, 0) z (0, 0, 1) at (-232, 0, 57)
copy_body "CopyPasteBodies14" bodies 10 9 11 8 makes body 12 makes body 13 makes body 14 makes body 15
move_body "Move49" bodies 12 13 14 15 to x (1, 0, 0) y (0, 1, 0) z (0, 0, 1) at (0, 0, -112)
move_body "Move50" bodies 6 5 4 7 to x (1, 0, 0) y (0, 1, 0) z (0, 0, 1) at (-138, 0, 0)
move_body "Move51" bodies 4 5 6 7 to x (1, 0, 0) y (0, 1, 0) z (0, 0, 1) at (1, 0, 0)
sketch "Sketch9" plane through (0, 0, 0) normal (0, 1, 0) x (1, 0, 0)
  circle A0 centre (0, 110) radius 32
  arc A1 (48.4482, 130.2242) -> (48.1066, 88.9762) centre (0, 110) ccw
  spline S0 degree 5 poles (48.1066, 88.9762) (48.2645, 89.3375) (48.5799, 90.043) (49.0515, 91.0499) (49.6862, 92.2877) (50.5348, 93.6491) (51.4896, 94.8133) (52.5876, 95.7778) (53.8333, 96.5585) (55.1674, 97.2091) (56.3365, 97.7434) (57.1616, 98.1776) (57.6822, 98.5123) (57.9641, 98.7213) (58.0483, 98.7867) knots -1 -1 -1 -1 -1 -1 -0.9 -0.8 -0.7 -0.6 -0.5 -0.4 -0.3 -0.2 -0.1 -0.055622 -0.055622 -0.055622 -0.055622 -0.055622 -0.055622
  arc A2 (58.0483, 98.7867) -> (60, 102.75) centre (55, 102.75) ccw
  line L0 (60, 102.75) -> (60, 117.25)
  arc A3 (60, 117.25) -> (57.9542, 121.2839) centre (55, 117.25) ccw
  spline S1 degree 5 poles (57.9542, 121.2839) (57.8883, 121.3329) (57.6234, 121.5231) (57.1228, 121.8387) (56.3243, 122.2559) (55.1846, 122.7765) (53.845, 123.4321) (52.5838, 124.2253) (51.463, 125.2079) (50.4859, 126.3894) (49.7057, 127.6326) (49.1456, 128.7074) (48.7586, 129.5278) (48.5283, 130.0423) (48.4482, 130.2242) knots 0.065909 0.065909 0.065909 0.065909 0.065909 0.065909 0.1 0.2 0.3 0.4 0.5 0.6 0.7 0.8 0.9 0.95371 0.95371 0.95371 0.95371 0.95371 0.95371
  line L1 (16.3, 112.2) -> (16.3, 95)
  arc A4 (16.3, 95) -> (17.8, 93.5) centre (17.8, 95) ccw
  line L2 (17.8, 93.5) -> (18, 93.5)
  arc A5 (18, 93.5) -> (22, 97.5) centre (18, 97.5) ccw
  line L3 (22, 97.5) -> (22, 129.5)
  spline S2 degree 2 poles (22, 129.5) (22, 134.5) (12, 134.5) knots 0 0 0 1 1 1
  spline S3 degree 2 poles (12, 134.5) (2, 134.5) (2, 129.5) knots -1 -1 -1 0 0 0
  line L4 (2, 129.5) -> (17, 129.5)
  line L5 (17, 129.5) -> (17, 126)
  line L6 (17, 126) -> (12, 126)
  line L7 (12, 126) -> (12, 121.5)
  line L8 (12, 121.5) -> (17, 121.5)
  line L9 (17, 121.5) -> (17, 118)
  line L10 (17, 118) -> (9.5, 118)
  line L11 (9.5, 118) -> (9.5, 114)
  arc A6 (9.5, 114) -> (10, 113.5) centre (10, 114) ccw
  spline S4 degree 5 poles (10, 113.5) (10.5, 113.5) (10.5, 114) (12.5, 114) (14.5, 114) (14.5, 113.5) (15, 113.5) knots 0 0 0 0 0 0 0.5 1 1 1 1 1 1
  arc A7 (16.3, 112.2) -> (15, 113.5) centre (15, 112.2) ccw
  line L12 (7.7, 109.8) -> (7.7, 127)
  arc A8 (7.7, 127) -> (6.2, 128.5) centre (6.2, 127) ccw
  line L13 (6.2, 128.5) -> (6, 128.5)
  arc A9 (6, 128.5) -> (2, 124.5) centre (6, 124.5) ccw
  line L14 (2, 124.5) -> (2, 92.5)
  spline S5 degree 2 poles (2, 92.5) (2, 87.5) (12, 87.5) knots 0 0 0 1 1 1
  spline S6 degree 2 poles (12, 87.5) (22, 87.5) (22, 92.5) knots -1 -1 -1 0 0 0
  line L15 (22, 92.5) -> (7, 92.5)
  line L16 (7, 92.5) -> (7, 96)
  line L17 (7, 96) -> (12, 96)
  line L18 (12, 96) -> (12, 100.5)
  line L19 (12, 100.5) -> (7, 100.5)
  line L20 (7, 100.5) -> (7, 104)
  line L21 (7, 104) -> (14.5, 104)
  line L22 (14.5, 104) -> (14.5, 108)
  arc A10 (14.5, 108) -> (14, 108.5) centre (14, 108) ccw
  spline S7 degree 5 poles (14, 108.5) (13.5, 108.5) (13.5, 108) (11.5, 108) (9.5, 108) (9.5, 108.5) (9, 108.5) knots 0 0 0 0 0 0 0.5 1 1 1 1 1 1
  arc A11 (7.7, 109.8) -> (9, 108.5) centre (9, 109.8) ccw
  line L23 (-6.7, 112.2) -> (-6.7, 95)
  arc A12 (-6.7, 95) -> (-5.2, 93.5) centre (-5.2, 95) ccw
  line L24 (-5.2, 93.5) -> (-5, 93.5)
  arc A13 (-5, 93.5) -> (-1, 97.5) centre (-5, 97.5) ccw
  line L25 (-1, 97.5) -> (-1, 129.5)
  spline S8 degree 2 poles (-1, 129.5) (-1, 134.5) (-11, 134.5) knots 0 0 0 1 1 1
  spline S9 degree 2 poles (-11, 134.5) (-21, 134.5) (-21, 129.5) knots -1 -1 -1 0 0 0
  line L26 (-21, 129.5) -> (-6, 129.5)
  line L27 (-6, 129.5) -> (-6, 126)
  line L28 (-6, 126) -> (-11, 126)
  line L29 (-11, 126) -> (-11, 121.5)
  line L30 (-11, 121.5) -> (-6, 121.5)
  line L31 (-6, 121.5) -> (-6, 118)
  line L32 (-6, 118) -> (-13.5, 118)
  line L33 (-13.5, 118) -> (-13.5, 114)
  arc A14 (-13.5, 114) -> (-13, 113.5) centre (-13, 114) ccw
  spline S10 degree 5 poles (-13, 113.5) (-12.5, 113.5) (-12.5, 114) (-10.5, 114) (-8.5, 114) (-8.5, 113.5) (-8, 113.5) knots 0 0 0 0 0 0 0.5 1 1 1 1 1 1
  arc A15 (-6.7, 112.2) -> (-8, 113.5) centre (-8, 112.2) ccw
  line L34 (-15.3, 109.8) -> (-15.3, 127)
  arc A16 (-15.3, 127) -> (-16.8, 128.5) centre (-16.8, 127) ccw
  line L35 (-16.8, 128.5) -> (-17, 128.5)
  arc A17 (-17, 128.5) -> (-21, 124.5) centre (-17, 124.5) ccw
  line L36 (-21, 124.5) -> (-21, 92.5)
  spline S11 degree 2 poles (-21, 92.5) (-21, 87.5) (-11, 87.5) knots 0 0 0 1 1 1
  spline S12 degree 2 poles (-11, 87.5) (-1, 87.5) (-1, 92.5) knots -1 -1 -1 0 0 0
  line L37 (-1, 92.5) -> (-16, 92.5)
  line L38 (-16, 92.5) -> (-16, 96)
  line L39 (-16, 96) -> (-11, 96)
  line L40 (-11, 96) -> (-11, 100.5)
  line L41 (-11, 100.5) -> (-16, 100.5)
  line L42 (-16, 100.5) -> (-16, 104)
  line L43 (-16, 104) -> (-8.5, 104)
  line L44 (-8.5, 104) -> (-8.5, 108)
  arc A18 (-8.5, 108) -> (-9, 108.5) centre (-9, 108) ccw
  spline S13 degree 5 poles (-9, 108.5) (-9.5, 108.5) (-9.5, 108) (-11.5, 108) (-13.5, 108) (-13.5, 108.5) (-14, 108.5) knots 0 0 0 0 0 0 0.5 1 1 1 1 1 1
  arc A19 (-15.3, 109.8) -> (-14, 108.5) centre (-14, 109.8) ccw
  arc A20 (44.5661, 27.751) -> (1.75, 52.4708) centre (0, 0) ccw
  circle A21 centre (0, 0) radius 32
  line L45 (-47.233, 5.4225) -> (-31.5336, 35.5808)
  arc A22 (-22.6499, 41.8012) -> (-31.5336, 35.5808) centre (0, 0) ccw
  line L46 (-22.6499, 41.8012) -> (11.0592, 46.2391)
  arc A23 (21.2501, 42.5299) -> (11.0592, 46.2391) centre (0, 0) ccw
  line L47 (21.2501, 42.5299) -> (44.2201, 17.4625)
  line L48 (44.2201, 17.4625) -> (38.5317, 12.25)
  line L49 (38.5317, 12.25) -> (34.8906, 12.25)
  line L50 (34.8906, 12.25) -> (13.5824, 35.5038)
  arc A24 (13.5824, 35.5038) -> (12.4167, 35.9281) centre (0, 0) ccw
  line L51 (12.4167, 35.9281) -> (-21.2925, 31.4902)
  arc A25 (-21.2925, 31.4902) -> (-22.3086, 30.7786) centre (0, 0) ccw
  line L52 (-22.3086, 30.7786) -> (-38.0081, 0.6203)
  arc A26 (-38.0081, 0.6203) -> (-38.0081, -0.6203) centre (0, 0) ccw
  line L53 (-38.0081, -0.6203) -> (-22.3086, -30.7786)
  arc A27 (-22.3086, -30.7786) -> (-21.2925, -31.4902) centre (0, 0) ccw
  line L54 (-21.2925, -31.4902) -> (12.4167, -35.9281)
  arc A28 (12.4167, -35.9281) -> (13.5824, -35.5038) centre (0, 0) ccw
  line L55 (13.5824, -35.5038) -> (36.5525, -10.4364)
  arc A29 (36.5525, -10.4364) -> (36.8706, -9.25) centre (0, 0) ccw
  line L56 (36.8706, -9.25) -> (34, -9.25)
  line L57 (34, -9.25) -> (34, 9.25)
  line L58 (34, 9.25) -> (57, 9.25)
  line L59 (57, 9.25) -> (57, 4.3983)
  line L60 (57, 4.3983) -> (60, 4.3983)
  line L61 (60, 4.3983) -> (60, 7.25)
  arc A30 (60, 7.25) -> (57.9542, 11.2839) centre (55, 7.25) ccw
  spline S14 degree 5 poles (57.9542, 11.2839) (57.8883, 11.3329) (57.6234, 11.5231) (57.1228, 11.8387) (56.3243, 12.2559) (55.1846, 12.7765) (53.845, 13.4321) (52.5838, 14.2253) (51.463, 15.2079) (50.4859, 16.3894) (49.7057, 17.6326) (49.1456, 18.7074) (48.7586, 19.5278) (48.5283, 20.0423) (48.4482, 20.2242) knots 0.065909 0.065909 0.065909 0.065909 0.065909 0.065909 0.1 0.2 0.3 0.4 0.5 0.6 0.7 0.8 0.9 0.95371 0.95371 0.95371 0.95371 0.95371 0.95371
  arc A31 (48.4482, 20.2242) -> (46.3161, 24.7199) centre (0, 0) ccw
  line L62 (46.3161, 24.7199) -> (42.0208, 22.24)
  arc A32 (42.0208, 22.24) -> (40.2708, 25.2711) centre (0, 0) ccw
  line L63 (40.2708, 25.2711) -> (44.5661, 27.751)
  arc A33 (44.5661, 27.751) -> (1.75, 52.4708) centre (0, 0) ccw
  line L64 (1.75, 52.4708) -> (1.75, 47.511)
  arc A34 (1.75, 47.511) -> (-1.75, 47.511) centre (0, 0) ccw
  line L65 (-1.75, 47.511) -> (-1.75, 52.4708)
  arc A35 (-1.75, 52.4708) -> (-44.5661, 27.751) centre (0, 0) ccw
  line L66 (-44.5661, 27.751) -> (-40.2708, 25.2711)
  arc A36 (-40.2708, 25.2711) -> (-42.0208, 22.24) centre (0, 0) ccw
  line L67 (-42.0208, 22.24) -> (-46.3161, 24.7199)
  arc A37 (-46.3161, 24.7199) -> (-46.3161, -24.7199) centre (0, 0) ccw
  line L68 (-46.3161, -24.7199) -> (-42.0208, -22.24)
  arc A38 (-42.0208, -22.24) -> (-40.2708, -25.2711) centre (0, 0) ccw
  line L69 (-40.2708, -25.2711) -> (-44.5661, -27.751)
  arc A39 (-44.5661, -27.751) -> (-1.75, -52.4708) centre (0, 0) ccw
  line L70 (-1.75, -52.4708) -> (-1.75, -47.511)
  arc A40 (-1.75, -47.511) -> (1.75, -47.511) centre (0, 0) ccw
  line L71 (1.75, -47.511) -> (1.75, -52.4708)
  arc A41 (1.75, -52.4708) -> (44.5661, -27.751) centre (0, 0) ccw
  line L72 (44.5661, -27.751) -> (40.2708, -25.2711)
  arc A42 (40.2708, -25.2711) -> (42.0208, -22.24) centre (0, 0) ccw
  line L73 (42.0208, -22.24) -> (46.3161, -24.7199)
  arc A43 (46.3161, -24.7199) -> (48.1066, -21.0238) centre (0, 0) ccw
  spline S15 degree 5 poles (48.1066, -21.0238) (48.2645, -20.6625) (48.5799, -19.957) (49.0515, -18.9501) (49.6862, -17.7123) (50.5348, -16.3509) (51.4896, -15.1867) (52.5876, -14.2222) (53.8333, -13.4415) (55.1674, -12.7909) (56.3365, -12.2566) (57.1616, -11.8224) (57.6822, -11.4877) (57.9641, -11.2787) (58.0483, -11.2133) knots -1 -1 -1 -1 -1 -1 -0.9 -0.8 -0.7 -0.6 -0.5 -0.4 -0.3 -0.2 -0.1 -0.055622 -0.055622 -0.055622 -0.055622 -0.055622 -0.055622
  arc A44 (58.0483, -11.2133) -> (60, -7.25) centre (55, -7.25) ccw
  line L74 (60, -7.25) -> (60, -4.6017)
  line L75 (60, -4.6017) -> (57, -4.6017)
  line L76 (57, -4.6017) -> (57, -9.25)
  spline S16 degree 5 poles (57, -9.25) (56.1534, -9.25) (54.916, -9.3573) (53.7693, -9.6287) (52.7064, -10.0415) (51.7204, -10.561) (51.3871, -10.7526) knots 0 0 0 0 0 0 0.2 0.306371 0.306371 0.306371 0.306371 0.306371 0.306371
  spline S17 degree 5 poles (51.3871, -10.7526) (51.0937, -10.9213) (50.1955, -11.4779) (48.7982, -12.541) (47.0834, -14.2002) (45.7147, -15.761) (44.8358, -16.7778) (44.4003, -17.2659) (44.2201, -17.4625) knots 0.306371 0.306371 0.306371 0.306371 0.306371 0.306371 0.4 0.6 0.8 1 1 1 1 1 1
  line L77 (44.2201, -17.4625) -> (21.2501, -42.5299)
  arc A45 (11.0592, -46.2391) -> (21.2501, -42.5299) centre (0, 0) ccw
  line L78 (11.0592, -46.2391) -> (-22.6499, -41.8012)
  arc A46 (-31.5336, -35.5808) -> (-22.6499, -41.8012) centre (0, 0) ccw
  line L79 (-31.5336, -35.5808) -> (-47.233, -5.4225)
  arc A47 (-47.233, 5.4225) -> (-47.233, -5.4225) centre (0, 0) ccw
  line L80 (16.3, 0.2) -> (16.3, -17)
  arc A48 (16.3, -17) -> (17.8, -18.5) centre (17.8, -17) ccw
  line L81 (17.8, -18.5) -> (18, -18.5)
  arc A49 (18, -18.5) -> (22, -14.5) centre (18, -14.5) ccw
  line L82 (22, -14.5) -> (22, 17.5)
  spline S18 degree 2 poles (22, 17.5) (22, 22.5) (12, 22.5) knots 0 0 0 1 1 1
  spline S19 degree 2 poles (12, 22.5) (2, 22.5) (2, 17.5) knots -1 -1 -1 0 0 0
  line L83 (2, 17.5) -> (17, 17.5)
  line L84 (17, 17.5) -> (17, 14)
  line L85 (17, 14) -> (12, 14)
  line L86 (12, 14) -> (12, 9.5)
  line L87 (12, 9.5) -> (17, 9.5)
  line L88 (17, 9.5) -> (17, 6)
  line L89 (17, 6) -> (9.5, 6)
  line L90 (9.5, 6) -> (9.5, 2)
  arc A50 (9.5, 2) -> (10, 1.5) centre (10, 2) ccw
  spline S20 degree 5 poles (10, 1.5) (10.5, 1.5) (10.5, 2) (12.5, 2) (14.5, 2) (14.5, 1.5) (15, 1.5) knots 0 0 0 0 0 0 0.5 1 1 1 1 1 1
  arc A51 (16.3, 0.2) -> (15, 1.5) centre (15, 0.2) ccw
  line L91 (7.7, -2.2) -> (7.7, 15)
  arc A52 (7.7, 15) -> (6.2, 16.5) centre (6.2, 15) ccw
  line L92 (6.2, 16.5) -> (6, 16.5)
  arc A53 (6, 16.5) -> (2, 12.5) centre (6, 12.5) ccw
  line L93 (2, 12.5) -> (2, -19.5)
  spline S21 degree 2 poles (2, -19.5) (2, -24.5) (12, -24.5) knots 0 0 0 1 1 1
  spline S22 degree 2 poles (12, -24.5) (22, -24.5) (22, -19.5) knots -1 -1 -1 0 0 0
  line L94 (22, -19.5) -> (7, -19.5)
  line L95 (7, -19.5) -> (7, -16)
  line L96 (7, -16) -> (12, -16)
  line L97 (12, -16) -> (12, -11.5)
  line L98 (12, -11.5) -> (7, -11.5)
  line L99 (7, -11.5) -> (7, -8)
  line L100 (7, -8) -> (14.5, -8)
  line L101 (14.5, -8) -> (14.5, -4)
  arc A54 (14.5, -4) -> (14, -3.5) centre (14, -4) ccw
  spline S23 degree 5 poles (14, -3.5) (13.5, -3.5) (13.5, -4) (11.5, -4) (9.5, -4) (9.5, -3.5) (9, -3.5) knots 0 0 0 0 0 0 0.5 1 1 1 1 1 1
  arc A55 (7.7, -2.2) -> (9, -3.5) centre (9, -2.2) ccw
  line L102 (-15.3, -2.2) -> (-15.3, 15)
  arc A56 (-15.3, 15) -> (-16.8, 16.5) centre (-16.8, 15) ccw
  line L103 (-16.8, 16.5) -> (-17, 16.5)
  arc A57 (-17, 16.5) -> (-21, 12.5) centre (-17, 12.5) ccw
  line L104 (-21, 12.5) -> (-21, -19.5)
  spline S24 degree 2 poles (-21, -19.5) (-21, -24.5) (-11, -24.5) knots 0 0 0 1 1 1
  spline S25 degree 2 poles (-11, -24.5) (-1, -24.5) (-1, -19.5) knots -1 -1 -1 0 0 0
  line L105 (-1, -19.5) -> (-16, -19.5)
  line L106 (-16, -19.5) -> (-16, -16)
  line L107 (-16, -16) -> (-11, -16)
  line L108 (-11, -16) -> (-11, -11.5)
  line L109 (-11, -11.5) -> (-16, -11.5)
  line L110 (-16, -11.5) -> (-16, -8)
  line L111 (-16, -8) -> (-8.5, -8)
  line L112 (-8.5, -8) -> (-8.5, -4)
  arc A58 (-8.5, -4) -> (-9, -3.5) centre (-9, -4) ccw
  spline S26 degree 5 poles (-9, -3.5) (-9.5, -3.5) (-9.5, -4) (-11.5, -4) (-13.5, -4) (-13.5, -3.5) (-14, -3.5) knots 0 0 0 0 0 0 0.5 1 1 1 1 1 1
  arc A59 (-15.3, -2.2) -> (-14, -3.5) centre (-14, -2.2) ccw
  line L113 (-6.7, 0.2) -> (-6.7, -17)
  arc A60 (-6.7, -17) -> (-5.2, -18.5) centre (-5.2, -17) ccw
  line L114 (-5.2, -18.5) -> (-5, -18.5)
  arc A61 (-5, -18.5) -> (-1, -14.5) centre (-5, -14.5) ccw
  line L115 (-1, -14.5) -> (-1, 17.5)
  spline S27 degree 2 poles (-1, 17.5) (-1, 22.5) (-11, 22.5) knots 0 0 0 1 1 1
  spline S28 degree 2 poles (-11, 22.5) (-21, 22.5) (-21, 17.5) knots -1 -1 -1 0 0 0
  line L116 (-21, 17.5) -> (-6, 17.5)
  line L117 (-6, 17.5) -> (-6, 14)
  line L118 (-6, 14) -> (-11, 14)
  line L119 (-11, 14) -> (-11, 9.5)
  line L120 (-11, 9.5) -> (-6, 9.5)
  line L121 (-6, 9.5) -> (-6, 6)
  line L122 (-6, 6) -> (-13.5, 6)
  line L123 (-13.5, 6) -> (-13.5, 2)
  arc A62 (-13.5, 2) -> (-13, 1.5) centre (-13, 2) ccw
  spline S29 degree 5 poles (-13, 1.5) (-12.5, 1.5) (-12.5, 2) (-10.5, 2) (-8.5, 2) (-8.5, 1.5) (-8, 1.5) knots 0 0 0 0 0 0 0.5 1 1 1 1 1 1
  arc A63 (-6.7, 0.2) -> (-8, 1.5) centre (-8, 0.2) ccw
  line L124 (84.1358, 91.228) -> (85.3627, 100.5476)
  line L125 (85.3627, 100.5476) -> (116.0975, 96.5013)
  line L126 (116.0975, 96.5013) -> (114.8705, 87.1817)
  line L127 (114.8705, 87.1817) -> (84.1358, 91.228)
  line L128 (80.0356, 89.7357) -> (59.0923, 66.8801)
  line L129 (59.0923, 66.8801) -> (52.1619, 73.2306)
  line L130 (52.1619, 73.2306) -> (73.1052, 96.0862)
  line L131 (73.1052, 96.0862) -> (80.0356, 89.7357)
  line L132 (118.4448, 84.679) -> (126.7827, 89.0194)
  line L133 (126.7827, 89.0194) -> (141.0969, 61.5221)
  line L134 (141.0969, 61.5221) -> (132.759, 57.1817)
  line L135 (132.759, 57.1817) -> (118.4448, 84.679)
  line L136 (80.0356, 20.2643) -> (73.1052, 13.9138)
  line L137 (73.1052, 13.9138) -> (52.1619, 36.7694)
  line L138 (52.1619, 36.7694) -> (59.0923, 43.1199)
  line L139 (59.0923, 43.1199) -> (80.0356, 20.2643)
  circle A64 centre (95, 55) radius 32
  line L140 (114.8705, 22.8183) -> (116.0975, 13.4987)
  line L141 (116.0975, 13.4987) -> (85.3627, 9.4524)
  line L142 (85.3627, 9.4524) -> (84.1358, 18.772)
  line L143 (84.1358, 18.772) -> (114.8705, 22.8183)
  line L144 (132.759, 52.8183) -> (141.0969, 48.4779)
  line L145 (141.0969, 48.4779) -> (126.7827, 20.9806)
  line L146 (126.7827, 20.9806) -> (118.4448, 25.321)
  line L147 (118.4448, 25.321) -> (132.759, 52.8183)
  line L148 (35, 59.6017) -> (45, 59.6017)
  line L149 (45, 59.6017) -> (45, 50.6017)
  line L150 (45, 50.6017) -> (35, 50.6017)
  line L151 (35, 50.6017) -> (35, 47.75)
  arc A65 (35, 47.75) -> (37.0458, 43.7161) centre (40, 47.75) ccw
  spline S30 degree 5 poles (37.0458, 43.7161) (37.1117, 43.6671) (37.3766, 43.4769) (37.8772, 43.1613) (38.6757, 42.7441) (39.8154, 42.2235) (41.155, 41.5679) (42.4162, 40.7747) (43.537, 39.7921) (44.5141, 38.6106) (45.2943, 37.3674) (45.8544, 36.2926) (46.2414, 35.4722) (46.4717, 34.9577) (46.5518, 34.7758) knots 0.065909 0.065909 0.065909 0.065909 0.065909 0.065909 0.1 0.2 0.3 0.4 0.5 0.6 0.7 0.8 0.9 0.95371 0.95371 0.95371 0.95371 0.95371 0.95371
  arc A66 (46.5518, 34.7758) -> (46.8934, 76.0238) centre (95, 55) ccw
  spline S31 degree 5 poles (46.8934, 76.0238) (46.7355, 75.6625) (46.4201, 74.957) (45.9485, 73.9501) (45.3138, 72.7123) (44.4652, 71.3509) (43.5104, 70.1867) (42.4124, 69.2222) (41.1667, 68.4415) (39.8326, 67.7909) (38.6635, 67.2566) (37.8384, 66.8224) (37.3178, 66.4877) (37.0359, 66.2787) (36.9517, 66.2133) knots -1 -1 -1 -1 -1 -1 -0.9 -0.8 -0.7 -0.6 -0.5 -0.4 -0.3 -0.2 -0.1 -0.055622 -0.055622 -0.055622 -0.055622 -0.055622 -0.055622
  arc A67 (36.9517, 66.2133) -> (35, 62.25) centre (40, 62.25) ccw
  line L152 (35, 62.25) -> (35, 59.6017)
  line L153 (88.3, 57.2) -> (88.3, 40)
  arc A68 (88.3, 40) -> (89.8, 38.5) centre (89.8, 40) ccw
  line L154 (89.8, 38.5) -> (90, 38.5)
  arc A69 (90, 38.5) -> (94, 42.5) centre (90, 42.5) ccw
  line L155 (94, 42.5) -> (94, 74.5)
  spline S32 degree 2 poles (94, 74.5) (94, 79.5) (84, 79.5) knots 0 0 0 1 1 1
  spline S33 degree 2 poles (84, 79.5) (74, 79.5) (74, 74.5) knots -1 -1 -1 0 0 0
  line L156 (74, 74.5) -> (89, 74.5)
  line L157 (89, 74.5) -> (89, 71)
  line L158 (89, 71) -> (84, 71)
  line L159 (84, 71) -> (84, 66.5)
  line L160 (84, 66.5) -> (89, 66.5)
  line L161 (89, 66.5) -> (89, 63)
  line L162 (89, 63) -> (81.5, 63)
  line L163 (81.5, 63) -> (81.5, 59)
  arc A70 (81.5, 59) -> (82, 58.5) centre (82, 59) ccw
  spline S34 degree 5 poles (82, 58.5) (82.5, 58.5) (82.5, 59) (84.5, 59) (86.5, 59) (86.5, 58.5) (87, 58.5) knots 0 0 0 0 0 0 0.5 1 1 1 1 1 1
  arc A71 (88.3, 57.2) -> (87, 58.5) centre (87, 57.2) ccw
  line L164 (79.7, 54.8) -> (79.7, 72)
  arc A72 (79.7, 72) -> (78.2, 73.5) centre (78.2, 72) ccw
  line L165 (78.2, 73.5) -> (78, 73.5)
  arc A73 (78, 73.5) -> (74, 69.5) centre (78, 69.5) ccw
  line L166 (74, 69.5) -> (74, 37.5)
  spline S35 degree 2 poles (74, 37.5) (74, 32.5) (84, 32.5) knots 0 0 0 1 1 1
  spline S36 degree 2 poles (84, 32.5) (94, 32.5) (94, 37.5) knots -1 -1 -1 0 0 0
  line L167 (94, 37.5) -> (79, 37.5)
  line L168 (79, 37.5) -> (79, 41)
  line L169 (79, 41) -> (84, 41)
  line L170 (84, 41) -> (84, 45.5)
  line L171 (84, 45.5) -> (79, 45.5)
  line L172 (79, 45.5) -> (79, 49)
  line L173 (79, 49) -> (86.5, 49)
  line L174 (86.5, 49) -> (86.5, 53)
  arc A74 (86.5, 53) -> (86, 53.5) centre (86, 53) ccw
  spline S37 degree 5 poles (86, 53.5) (85.5, 53.5) (85.5, 53) (83.5, 53) (81.5, 53) (81.5, 53.5) (81, 53.5) knots 0 0 0 0 0 0 0.5 1 1 1 1 1 1
  arc A75 (79.7, 54.8) -> (81, 53.5) centre (81, 54.8) ccw
  line L175 (97, 69.5) -> (97, 37.5)
  line L176 (102.7, 54.8) -> (102.7, 72)
  arc A76 (102.7, 72) -> (101.2, 73.5) centre (101.2, 72) ccw
  line L177 (101.2, 73.5) -> (101, 73.5)
  arc A77 (101, 73.5) -> (97, 69.5) centre (101, 69.5) ccw
  line L178 (97, 69.5) -> (97, 37.5)
  spline S38 degree 2 poles (97, 37.5) (97, 32.5) (107, 32.5) knots 0 0 0 1 1 1
  spline S39 degree 2 poles (107, 32.5) (117, 32.5) (117, 37.5) knots -1 -1 -1 0 0 0
  line L179 (117, 37.5) -> (102, 37.5)
  line L180 (102, 37.5) -> (102, 41)
  line L181 (102, 41) -> (107, 41)
  line L182 (107, 41) -> (107, 45.5)
  line L183 (107, 45.5) -> (102, 45.5)
  line L184 (102, 45.5) -> (102, 49)
  line L185 (102, 49) -> (109.5, 49)
  line L186 (109.5, 49) -> (109.5, 53)
  arc A78 (109.5, 53) -> (109, 53.5) centre (109, 53) ccw
  spline S40 degree 5 poles (109, 53.5) (108.5, 53.5) (108.5, 53) (106.5, 53) (104.5, 53) (104.5, 53.5) (104, 53.5) knots 0 0 0 0 0 0 0.5 1 1 1 1 1 1
  arc A79 (102.7, 54.8) -> (104, 53.5) centre (104, 54.8) ccw
  line L187 (111.3, 57.2) -> (111.3, 40)
  arc A80 (111.3, 40) -> (112.8, 38.5) centre (112.8, 40) ccw
  line L188 (112.8, 38.5) -> (113, 38.5)
  arc A81 (113, 38.5) -> (117, 42.5) centre (113, 42.5) ccw
  line L189 (117, 42.5) -> (117, 74.5)
  spline S41 degree 2 poles (117, 74.5) (117, 79.5) (107, 79.5) knots 0 0 0 1 1 1
  spline S42 degree 2 poles (107, 79.5) (97, 79.5) (97, 74.5) knots -1 -1 -1 0 0 0
  line L190 (97, 74.5) -> (112, 74.5)
  line L191 (112, 74.5) -> (112, 71)
  line L192 (112, 71) -> (107, 71)
  line L193 (107, 71) -> (107, 66.5)
  line L194 (107, 66.5) -> (112, 66.5)
  line L195 (112, 66.5) -> (112, 63)
  line L196 (112, 63) -> (104.5, 63)
  line L197 (104.5, 63) -> (104.5, 59)
  arc A82 (104.5, 59) -> (105, 58.5) centre (105, 59) ccw
  spline S43 degree 5 poles (105, 58.5) (105.5, 58.5) (105.5, 59) (107.5, 59) (109.5, 59) (109.5, 58.5) (110, 58.5) knots 0 0 0 0 0 0 0.5 1 1 1 1 1 1
  arc A83 (111.3, 57.2) -> (110, 58.5) centre (110, 57.2) ccw
  point P0 (17, 6)
  point P1 (102, 49)
extrude "Extrude1" [suppressed]
delete_body "RemoveBody1" bodies 16
delete_body "RemoveBody2" bodies 17
extrude "Extrude3" [suppressed]
move_body "Move2" [suppressed]
moveface "MoveFace1" [suppressed]
move_body "Move4" [suppressed]
move_body "Move6" [suppressed]
extrude "Extrude5" [suppressed]
move_body "Move7" [suppressed]
extrude "Extrude6" [suppressed]
move_body "Move8" [suppressed]
move_body "Move9" [suppressed]
extrude "Extrude7" [suppressed]
copy_body "CopyPasteBodies1" [suppressed]
move_body "Move10" [suppressed]
move_body "Move11" [suppressed]
copy_body "CopyPasteBodies2" [suppressed]
move_body "Move12" [suppressed]
move_body "Move13" [suppressed]
copy_body "CopyPasteBodies3" [suppressed]
move_body "Move14" [suppressed]
copy_body "CopyPasteBodies4" [suppressed]
move_body "Move15" [suppressed]
move_body "Move16" [suppressed]